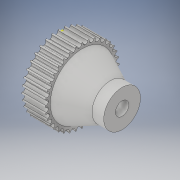
# Autodesk Inventor part: WheelGear
Saved by Autodesk Inventor 2018 (Build 220112000, 112)
## iProperties
Created: 2019-06-11
Part Number: WheelGear
Material: Generic
Document SubType Name: Modeling
Designer: anirudh
Density: 1 g/cm^3
Appearance: Default
Author: anirudh
Autodesk Inventor part; units mm, degrees
ref_plane "YZ Plane" through (0, 0, 0) normal (1, 0, 0) x (0, 1, 0)
ref_plane "XZ Plane" through (0, 0, 0) normal (0, 1, 0) x (-1, 0, 0)
ref_plane "XY Plane" through (0, 0, 0) normal (0, 0, 1) x (1, 0, 0)
sketch "Sketch2" plane through (0, 0, 0) normal (1, 0, 0) x (0, 1, 0)
  arc A0 (20.1957, 1.6009) -> (21.7494, 0.4688) centre (21.643, 1.955) ccw
  arc A1 (21.7494, -0.4688) -> (20.1957, -1.6009) centre (21.643, -1.955) ccw
  arc A2 (21.7494, -0.4688) -> (21.7494, 0.4688) centre (21.783, 0) ccw
  arc A3 (19.6109, 5.0835) -> (21.3376, 4.2384) centre (20.9747, 5.6836) ccw
  arc A4 (21.5004, 3.3151) -> (21.3376, 4.2384) centre (21.4521, 3.7826) ccw
  arc A5 (21.5004, 3.3151) -> (20.1669, 1.9304) centre (21.6537, 1.833) ccw
  arc A6 (18.4302, 8.4117) -> (20.2774, 7.8793) centre (19.6691, 9.2394) ccw
  arc A7 (20.5981, 6.9982) -> (20.2774, 7.8793) centre (20.4693, 7.4502) ccw
  arc A8 (20.5981, 6.9982) -> (19.5253, 5.403) centre (21.0064, 5.5652) ccw
  arc A9 (16.6895, 11.4842) -> (18.6011, 11.2807) centre (17.7659, 12.5146) ccw
  arc A10 (19.07, 10.4687) -> (18.6011, 11.2807) centre (18.8646, 10.8915) ccw
  arc A11 (19.07, 10.4687) -> (18.2904, 8.7114) centre (19.7209, 9.1284) ccw
  arc A12 (14.4418, 14.2079) -> (16.3597, 14.3394) centre (15.3228, 15.4095) ccw
  arc A13 (16.9624, 13.6211) -> (16.3597, 14.3394) centre (16.6867, 14.0018) ccw
  arc A14 (16.9624, 13.6211) -> (16.4998, 11.7552) centre (17.8361, 12.4142) ccw
  arc A15 (11.7552, 16.4998) -> (13.6211, 16.9624) centre (12.4142, 17.8361) ccw
  arc A16 (14.3394, 16.3597) -> (13.6211, 16.9624) centre (14.0018, 16.6867) ccw
  arc A17 (14.3394, 16.3597) -> (14.2079, 14.4418) centre (15.4095, 15.3228) ccw
  arc A18 (8.7114, 18.2904) -> (10.4687, 19.07) centre (9.1284, 19.7209) ccw
  arc A19 (11.2807, 18.6011) -> (10.4687, 19.07) centre (10.8915, 18.8646) ccw
  arc A20 (11.2807, 18.6011) -> (11.4842, 16.6895) centre (12.5146, 17.7659) ccw
  arc A21 (5.403, 19.5253) -> (6.9982, 20.5981) centre (5.5652, 21.0064) ccw
  arc A22 (7.8793, 20.2774) -> (6.9982, 20.5981) centre (7.4502, 20.4693) ccw
  arc A23 (7.8793, 20.2774) -> (8.4117, 18.4302) centre (9.2394, 19.6691) ccw
  arc A24 (1.9304, 20.1669) -> (3.3151, 21.5004) centre (1.833, 21.6537) ccw
  arc A25 (4.2384, 21.3376) -> (3.3151, 21.5004) centre (3.7826, 21.4521) ccw
  arc A26 (4.2384, 21.3376) -> (5.0835, 19.6109) centre (5.6836, 20.9747) ccw
  arc A27 (-1.6009, 20.1957) -> (-0.4688, 21.7494) centre (-1.955, 21.643) ccw
  arc A28 (0.4688, 21.7494) -> (-0.4688, 21.7494) centre (0, 21.783) ccw
  arc A29 (0.4688, 21.7494) -> (1.6009, 20.1957) centre (1.955, 21.643) ccw
  arc A30 (-5.0835, 19.6109) -> (-4.2384, 21.3376) centre (-5.6836, 20.9747) ccw
  arc A31 (-3.3151, 21.5004) -> (-4.2384, 21.3376) centre (-3.7826, 21.4521) ccw
  arc A32 (-3.3151, 21.5004) -> (-1.9304, 20.1669) centre (-1.833, 21.6537) ccw
  arc A33 (-8.4117, 18.4302) -> (-7.8793, 20.2774) centre (-9.2394, 19.6691) ccw
  arc A34 (-6.9982, 20.5981) -> (-7.8793, 20.2774) centre (-7.4502, 20.4693) ccw
  arc A35 (-6.9982, 20.5981) -> (-5.403, 19.5253) centre (-5.5652, 21.0064) ccw
  arc A36 (-11.4842, 16.6895) -> (-11.2807, 18.6011) centre (-12.5146, 17.7659) ccw
  arc A37 (-10.4687, 19.07) -> (-11.2807, 18.6011) centre (-10.8915, 18.8646) ccw
  arc A38 (-10.4687, 19.07) -> (-8.7114, 18.2904) centre (-9.1284, 19.7209) ccw
  arc A39 (-14.2079, 14.4418) -> (-14.3394, 16.3597) centre (-15.4095, 15.3228) ccw
  arc A40 (-13.6211, 16.9624) -> (-14.3394, 16.3597) centre (-14.0018, 16.6867) ccw
  arc A41 (-13.6211, 16.9624) -> (-11.7552, 16.4998) centre (-12.4142, 17.8361) ccw
  arc A42 (-16.4998, 11.7552) -> (-16.9624, 13.6211) centre (-17.8361, 12.4142) ccw
  arc A43 (-16.3597, 14.3394) -> (-16.9624, 13.6211) centre (-16.6867, 14.0018) ccw
  arc A44 (-16.3597, 14.3394) -> (-14.4418, 14.2079) centre (-15.3228, 15.4095) ccw
  arc A45 (-18.2904, 8.7114) -> (-19.07, 10.4687) centre (-19.7209, 9.1284) ccw
  arc A46 (-18.6011, 11.2807) -> (-19.07, 10.4687) centre (-18.8646, 10.8915) ccw
  arc A47 (-18.6011, 11.2807) -> (-16.6895, 11.4842) centre (-17.7659, 12.5146) ccw
  arc A48 (-19.5253, 5.403) -> (-20.5981, 6.9982) centre (-21.0064, 5.5652) ccw
  arc A49 (-20.2774, 7.8793) -> (-20.5981, 6.9982) centre (-20.4693, 7.4502) ccw
  arc A50 (-20.2774, 7.8793) -> (-18.4302, 8.4117) centre (-19.6691, 9.2394) ccw
  arc A51 (-20.1669, 1.9304) -> (-21.5004, 3.3151) centre (-21.6537, 1.833) ccw
  arc A52 (-21.3376, 4.2384) -> (-21.5004, 3.3151) centre (-21.4521, 3.7826) ccw
  arc A53 (-21.3376, 4.2384) -> (-19.6109, 5.0835) centre (-20.9747, 5.6836) ccw
  arc A54 (-20.1957, -1.6009) -> (-21.7494, -0.4688) centre (-21.643, -1.955) ccw
  arc A55 (-21.7494, 0.4688) -> (-21.7494, -0.4688) centre (-21.783, 0) ccw
  arc A56 (-21.7494, 0.4688) -> (-20.1957, 1.6009) centre (-21.643, 1.955) ccw
  arc A57 (-19.6109, -5.0835) -> (-21.3376, -4.2384) centre (-20.9747, -5.6836) ccw
  arc A58 (-21.5004, -3.3151) -> (-21.3376, -4.2384) centre (-21.4521, -3.7826) ccw
  arc A59 (-21.5004, -3.3151) -> (-20.1669, -1.9304) centre (-21.6537, -1.833) ccw
  arc A60 (-18.4302, -8.4117) -> (-20.2774, -7.8793) centre (-19.6691, -9.2394) ccw
  arc A61 (-20.5981, -6.9982) -> (-20.2774, -7.8793) centre (-20.4693, -7.4502) ccw
  arc A62 (-20.5981, -6.9982) -> (-19.5253, -5.403) centre (-21.0064, -5.5652) ccw
  arc A63 (-16.6895, -11.4842) -> (-18.6011, -11.2807) centre (-17.7659, -12.5146) ccw
  arc A64 (-19.07, -10.4687) -> (-18.6011, -11.2807) centre (-18.8646, -10.8915) ccw
  arc A65 (-19.07, -10.4687) -> (-18.2904, -8.7114) centre (-19.7209, -9.1284) ccw
  arc A66 (-14.4418, -14.2079) -> (-16.3597, -14.3394) centre (-15.3228, -15.4095) ccw
  arc A67 (-16.9624, -13.6211) -> (-16.3597, -14.3394) centre (-16.6867, -14.0018) ccw
  arc A68 (-16.9624, -13.6211) -> (-16.4998, -11.7552) centre (-17.8361, -12.4142) ccw
  arc A69 (-11.7552, -16.4998) -> (-13.6211, -16.9624) centre (-12.4142, -17.8361) ccw
  arc A70 (-14.3394, -16.3597) -> (-13.6211, -16.9624) centre (-14.0018, -16.6867) ccw
  arc A71 (-14.3394, -16.3597) -> (-14.2079, -14.4418) centre (-15.4095, -15.3228) ccw
  arc A72 (-8.7114, -18.2904) -> (-10.4687, -19.07) centre (-9.1284, -19.7209) ccw
  arc A73 (-11.2807, -18.6011) -> (-10.4687, -19.07) centre (-10.8915, -18.8646) ccw
  arc A74 (-11.2807, -18.6011) -> (-11.4842, -16.6895) centre (-12.5146, -17.7659) ccw
  arc A75 (-5.403, -19.5253) -> (-6.9982, -20.5981) centre (-5.5652, -21.0064) ccw
  arc A76 (-7.8793, -20.2774) -> (-6.9982, -20.5981) centre (-7.4502, -20.4693) ccw
  arc A77 (-7.8793, -20.2774) -> (-8.4117, -18.4302) centre (-9.2394, -19.6691) ccw
  arc A78 (-1.9304, -20.1669) -> (-3.3151, -21.5004) centre (-1.833, -21.6537) ccw
  arc A79 (-4.2384, -21.3376) -> (-3.3151, -21.5004) centre (-3.7826, -21.4521) ccw
  arc A80 (-4.2384, -21.3376) -> (-5.0835, -19.6109) centre (-5.6836, -20.9747) ccw
  arc A81 (1.6009, -20.1957) -> (0.4688, -21.7494) centre (1.955, -21.643) ccw
  arc A82 (-0.4688, -21.7494) -> (0.4688, -21.7494) centre (0, -21.783) ccw
  arc A83 (-0.4688, -21.7494) -> (-1.6009, -20.1957) centre (-1.955, -21.643) ccw
  arc A84 (5.0835, -19.6109) -> (4.2384, -21.3376) centre (5.6836, -20.9747) ccw
  arc A85 (3.3151, -21.5004) -> (4.2384, -21.3376) centre (3.7826, -21.4521) ccw
  arc A86 (3.3151, -21.5004) -> (1.9304, -20.1669) centre (1.833, -21.6537) ccw
  arc A87 (8.4117, -18.4302) -> (7.8793, -20.2774) centre (9.2394, -19.6691) ccw
  arc A88 (6.9982, -20.5981) -> (7.8793, -20.2774) centre (7.4502, -20.4693) ccw
  arc A89 (6.9982, -20.5981) -> (5.403, -19.5253) centre (5.5652, -21.0064) ccw
  arc A90 (11.4842, -16.6895) -> (11.2807, -18.6011) centre (12.5146, -17.7659) ccw
  arc A91 (10.4687, -19.07) -> (11.2807, -18.6011) centre (10.8915, -18.8646) ccw
  arc A92 (10.4687, -19.07) -> (8.7114, -18.2904) centre (9.1284, -19.7209) ccw
  arc A93 (14.2079, -14.4418) -> (14.3394, -16.3597) centre (15.4095, -15.3228) ccw
  arc A94 (13.6211, -16.9624) -> (14.3394, -16.3597) centre (14.0018, -16.6867) ccw
  arc A95 (13.6211, -16.9624) -> (11.7552, -16.4998) centre (12.4142, -17.8361) ccw
  arc A96 (16.4998, -11.7552) -> (16.9624, -13.6211) centre (17.8361, -12.4142) ccw
  arc A97 (16.3597, -14.3394) -> (16.9624, -13.6211) centre (16.6867, -14.0018) ccw
  arc A98 (16.3597, -14.3394) -> (14.4418, -14.2079) centre (15.3228, -15.4095) ccw
  arc A99 (18.2904, -8.7114) -> (19.07, -10.4687) centre (19.7209, -9.1284) ccw
  arc A100 (18.6011, -11.2807) -> (19.07, -10.4687) centre (18.8646, -10.8915) ccw
  arc A101 (18.6011, -11.2807) -> (16.6895, -11.4842) centre (17.7659, -12.5146) ccw
  arc A102 (19.5253, -5.403) -> (20.5981, -6.9982) centre (21.0064, -5.5652) ccw
  arc A103 (20.2774, -7.8793) -> (20.5981, -6.9982) centre (20.4693, -7.4502) ccw
  arc A104 (20.2774, -7.8793) -> (18.4302, -8.4117) centre (19.6691, -9.2394) ccw
  arc A105 (20.1669, -1.9304) -> (21.5004, -3.3151) centre (21.6537, -1.833) ccw
  arc A106 (21.3376, -4.2384) -> (21.5004, -3.3151) centre (21.4521, -3.7826) ccw
  arc A107 (21.3376, -4.2384) -> (19.6109, -5.0835) centre (20.9747, -5.6836) ccw
  arc A108 (20.1669, -1.9304) -> (20.1957, -1.6009) centre (0, 0) ccw
  arc A109 (20.1957, 1.6009) -> (20.1669, 1.9304) centre (0, 0) ccw
  arc A110 (19.6109, 5.0835) -> (19.5253, 5.403) centre (0, 0) ccw
  arc A111 (18.4302, 8.4117) -> (18.2904, 8.7114) centre (0, 0) ccw
  arc A112 (16.6895, 11.4842) -> (16.4998, 11.7552) centre (0, 0) ccw
  arc A113 (14.4418, 14.2079) -> (14.2079, 14.4418) centre (0, 0) ccw
  arc A114 (11.7552, 16.4998) -> (11.4842, 16.6895) centre (0, 0) ccw
  arc A115 (8.7114, 18.2904) -> (8.4117, 18.4302) centre (0, 0) ccw
  arc A116 (5.403, 19.5253) -> (5.0835, 19.6109) centre (0, 0) ccw
  arc A117 (1.9304, 20.1669) -> (1.6009, 20.1957) centre (0, 0) ccw
  arc A118 (-1.6009, 20.1957) -> (-1.9304, 20.1669) centre (0, 0) ccw
  arc A119 (-5.0835, 19.6109) -> (-5.403, 19.5253) centre (0, 0) ccw
  arc A120 (-8.4117, 18.4302) -> (-8.7114, 18.2904) centre (0, 0) ccw
  arc A121 (-11.4842, 16.6895) -> (-11.7552, 16.4998) centre (0, 0) ccw
  arc A122 (-14.2079, 14.4418) -> (-14.4418, 14.2079) centre (0, 0) ccw
  arc A123 (-16.4998, 11.7552) -> (-16.6895, 11.4842) centre (0, 0) ccw
  arc A124 (-18.2904, 8.7114) -> (-18.4302, 8.4117) centre (0, 0) ccw
  arc A125 (-19.5253, 5.403) -> (-19.6109, 5.0835) centre (0, 0) ccw
  arc A126 (-20.1669, 1.9304) -> (-20.1957, 1.6009) centre (0, 0) ccw
  arc A127 (-20.1957, -1.6009) -> (-20.1669, -1.9304) centre (0, 0) ccw
  arc A128 (-19.6109, -5.0835) -> (-19.5253, -5.403) centre (0, 0) ccw
  arc A129 (-18.4302, -8.4117) -> (-18.2904, -8.7114) centre (0, 0) ccw
  arc A130 (-16.6895, -11.4842) -> (-16.4998, -11.7552) centre (0, 0) ccw
  arc A131 (-14.4418, -14.2079) -> (-14.2079, -14.4418) centre (0, 0) ccw
  arc A132 (-11.7552, -16.4998) -> (-11.4842, -16.6895) centre (0, 0) ccw
  arc A133 (-8.7114, -18.2904) -> (-8.4117, -18.4302) centre (0, 0) ccw
  arc A134 (-5.403, -19.5253) -> (-5.0835, -19.6109) centre (0, 0) ccw
  arc A135 (-1.9304, -20.1669) -> (-1.6009, -20.1957) centre (0, 0) ccw
  arc A136 (1.6009, -20.1957) -> (1.9304, -20.1669) centre (0, 0) ccw
  arc A137 (5.0835, -19.6109) -> (5.403, -19.5253) centre (0, 0) ccw
  arc A138 (8.4117, -18.4302) -> (8.7114, -18.2904) centre (0, 0) ccw
  arc A139 (11.4842, -16.6895) -> (11.7552, -16.4998) centre (0, 0) ccw
  arc A140 (14.2079, -14.4418) -> (14.4418, -14.2079) centre (0, 0) ccw
  arc A141 (16.4998, -11.7552) -> (16.6895, -11.4842) centre (0, 0) ccw
  arc A142 (18.2904, -8.7114) -> (18.4302, -8.4117) centre (0, 0) ccw
  arc A143 (19.5253, -5.403) -> (19.6109, -5.0835) centre (0, 0) ccw
  point P0 (20.22, 1.6009)
  point P1 (22.253, 0)
  dimension "d13" = 360
  constraints: 216 point on circle, 108 centre point, 1 tangent, 469 other
extrude "Extrusion1" add sketch "Sketch2" along normal blind 12 and the other way blind 2
sketch "Sketch5" plane through (12, 0, 0) normal (1, 0, 0) x (0, 0, -1)
  circle A0 centre (0, 0) radius 11.43
  dimension "d20" = 22.86
  constraints: 1 centre point, 1 coincident
  measures "d20" diameter of A0
extrude "Extrusion3" cut sketch "Sketch5" against normal blind 12
ref_plane "Work Plane1" through (28.9164, 0, 0) normal (1, 0, 0) x (0, 0, -1)
sketch "Sketch6" plane through (28.9164, 0, 0) normal (1, 0, 0) x (0, 0, -1)
  circle A0 centre (0, 0) radius 4.0132
  circle A1 centre (0, 0) radius 11
  dimension "d24" = 8.0264
  dimension "d25" = 22
  constraints: 2 centre point, 2 coincident
  measures "d24" diameter of A0
  measures "d25" diameter of A1
extrude "Extrusion4" add sketch "Sketch6" along normal blind 7.0104
sketch "Sketch8" plane through (28.9164, 0, 0) normal (-1, 0, 0) x (0, 0, 1)
  circle A0 centre (0, 0) radius 9.525
  circle A1 centre (0, 0) radius 11
  dimension "d33" = 19.05
  constraints: 2 centre point, 2 coincident
  measures "d33" diameter of A0
extrude "Extrusion5" add sketch "Sketch8" along normal blind 6.985
sketch "Sketch9" plane through (0, 0, 0) normal (0, 0, 1) x (1, 0, 0)
  line L0 (12, -0.47) -> (12, 0.47) projected
  line L1 (12, 13.6211) -> (12, 11.7552) projected
  line L2 (21.9314, 11) -> (35.9268, 11) projected
  line L3 (12, 11.43) -> (12, 19.05)
  line L4 (21.9314, 11) -> (21.9314, -11) projected
  line L5 (21.9314, 11) -> (28.9164, 11)
  line L6 (12, 19.07) -> (-2, 19.07) projected
  line L7 (28.9164, 11) -> (12, 19.07)
  line L8 (12, 11.43) -> (12, -11.43) projected
  line L9 (12, 11.43) -> (21.9314, 11)
  line L10 (12, 19.07) -> (12, 11.43)
  line L11 (12, 11.43) -> (21.9314, 11)
  line L12 (21.9314, 11) -> (28.9164, 11)
  line L13 (28.9164, 11) -> (12, 19.07)
  line L14 (-7.1854, 0) -> (43.1122, 0) projected
  point P0 (0, 0)
  point P1 (12, 0.4688)
  point P2 (12, -0.4688)
  dimension "d40" = 6.985
  constraints: 16 end point, 2 point on line, 1 collinear, 1 perpendicular, 1 vertical
  measures "d40" distance of L2.start L5.end
revolve "Revolution1" add sketch "Sketch9" angle 360 about axis through (12, 0, 0) along (1, 0, 0) contours L3 L1 L10 L7 L2 L9
body "Solid1"
